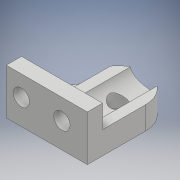
# Autodesk Inventor part: lower_deck_shaft_mount_v4_for_AD
Saved by Autodesk Inventor 2018.2 (Build 222227000, 227)
## iProperties
Created: 2017-08-21
Part Number: lower_deck_shaft_mount_v4_for_AD
Material: Generic
Document SubType Name: Modeling
Designer: ndz
Density: 1 g/cm^3
Appearance: Default
Author: ndz
Autodesk Inventor part; units mm, degrees
ref_plane "YZ Plane" through (0, 0, 0) normal (1, 0, 0) x (0, 1, 0)
ref_plane "XZ Plane" through (0, 0, 0) normal (0, 1, 0) x (-1, 0, 0)
ref_plane "XY Plane" through (0, 0, 0) normal (0, 0, 1) x (1, 0, 0)
sketch "Sketch1" plane through (0, 0, 0) normal (0, 0, 1) x (1, 0, 0)
  circle A0 centre (12.5, 11.5) radius 1.6
  line L0 (0, 0) -> (18, 0)
  line L1 (0, 0) -> (0, 3)
  arc A1 (18, 11.5) -> (7.7369, 14.25) centre (12.5, 11.5) ccw
  line L2 (12.5, 11.5) -> (7.7369, 14.25) construction
  line L3 (12.5, 11.5) -> (18, 11.5) construction
  line L4 (7.7369, 14.25) -> (0, 3)
  line L5 (18, 11.5) -> (18, 0)
  dimension "d17" = 3
  dimension "d19" = 11.5
  dimension "d23" = 90
  dimension "d25" = 12.5
  dimension "d31" = 5.5
  dimension "d32" = 150
  dimension "d49" = 3.2
  constraints: 13 end point, 2 centre point, 2 point on circle, 1 coincident, 1 horizontal, 1 parallel, 1 perpendicular, 1 tangent
  measures "d17" distance of L0.start L1.end
  measures "d19" distance from line of A0.centre L0
  measures "d23" angle of L0 L1
  measures "d25" distance from line of L1 A0.centre
  measures "d31" radius of A1
  measures "d32" angle of L3 L2
  measures "d49" diameter of A0
extrude "Extrusion1" add sketch "Sketch1" along normal blind 4.5
sketch "Sketch4" plane through (0, 0, 4.5) normal (0, 0, 1) x (1, 0, 0)
  line L0 (0, 3) -> (0, 0) projected
  line L1 (18, 0) -> (18, 3)
  line L2 (0, 0) -> (18, 0)
  line L3 (18, 0) -> (18, 3)
  line L4 (18, 3) -> (0, 3)
  line L5 (0, 3) -> (0, 0)
  line L6 (18, 0) -> (18, 11.5) projected
  constraints: 10 end point, 3 perpendicular, 1 collinear
extrude "Extrusion2" add sketch "Sketch4" along normal blind 4.5
sketch "Sketch5" plane through (0, 0, 0) normal (0, -1, 0) x (1, 0, 0)
  circle A0 centre (5, 5) radius 1.6
  circle A1 centre (13, 5) radius 1.6
  line L0 (0, 0) -> (18, 0) projected
  point P0 (20.0001, 0)
  dimension "d13" = 3.2
  dimension "d14" = 3.2
  dimension "d38" = 5
  dimension "d39" = 5
  dimension "d50" = 8
  constraints: 2 centre point
  measures "d13" diameter of A0
  measures "d14" diameter of A1
  measures "d38" distance from line of L0 A0.centre
  measures "d39" distance from line of L0 A1.centre
  measures "d50" distance of A1.centre A0.centre
extrude "Extrusion3" cut sketch "Sketch5" against normal through all
sketch "Sketch6" plane through (0, 3, 9) normal (0, 1, 0) x (1, 0, 0)
  circle A0 centre (5, 4) radius 1.6 projected
  circle A1 centre (5, 4) radius 3
  circle A2 centre (13, 4) radius 1.6 projected
  circle A3 centre (13, 4) radius 3
  line L0 (0, 9) -> (18, 9) projected
  point P0 (20.0001, 9)
  dimension "d34" = 6
  dimension "d35" = 6
  dimension "d40" = 5
  dimension "d41" = 5
  constraints: 2 centre point, 2 coincident
  measures "d34" diameter of A1
  measures "d35" diameter of A3
  measures "d40" distance from line of L0 A1.centre
  measures "d41" distance from line of L0 A3.centre
extrude "Extrusion4" cut sketch "Sketch6" along normal up to next
sketch "Sketch7" plane through (0, 0, 0) normal (0, -1, 0) x (1, 0, 0)
  line L0 (0, 0) -> (0, 9) projected
  line L1 (2.042, 0) -> (0, 0)
  line L2 (0, 0) -> (0, 9)
  line L3 (0, 9) -> (2.042, 9)
  line L4 (2.042, 9) -> (2.042, 0)
  constraints: 8 end point, 2 parallel, 1 horizontal, 1 perpendicular
extrude "Extrusion5" cut sketch "Sketch7" against normal up to next
body "Solid1"
